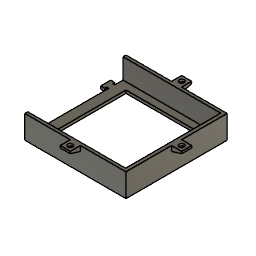
uC podstawa (Autodesk Fusion 360 design; units mm, degrees)
Autodesk Fusion 360 part; units mm, degrees
sketch "Szkic1" plane through (0, 0, 0) normal (0, 0, 1) x (1, 0, 0)
  line L0 (0, 0) -> (100, 0)
  line L1 (100, 0) -> (100, 100)
  line L2 (100, 100) -> (0, 100)
  line L3 (0, 100) -> (0, 0)
  dimension "d1" = 100
  dimension "d2" = 100
  constraint horizontal L0
  constraint vertical L1
  constraint horizontal L2
  constraint vertical L3
  constraint coincident L0.start L3.end
  measures "d1" distance of L0.start L0.end
  measures "d2" distance of L0.start L2.end
extrude "Wyciągnięcie proste1" add sketch "Szkic1" along normal blind 3
sketch "Szkic2" plane through (0, 0, 3) normal (0, 0, 1) x (-1, 0, 0)
  line L0 (0, -100) -> (0, 0)
  line L1 (0, 0) -> (-100, 0)
  line L2 (-100, 0) -> (-100, -100)
  line L3 (-100, -100) -> (0, -100)
  line L4 (-10, -10) -> (-90, -10)
  line L5 (-90, -10) -> (-90, -90)
  line L6 (-90, -90) -> (-10, -90)
  line L7 (-10, -90) -> (-10, -10)
  constraint horizontal L4
  constraint vertical L5
  constraint horizontal L6
  constraint vertical L7
extrude "Wyciągnięcie proste2" cut sketch "Szkic2" against normal blind 3 contours L4 L5 L6 L7
sketch "Szkic3" plane through (0, 0, 3) normal (0, 0, 1) x (-1, 0, 0)
  line L0 (-90, -10) -> (-10, -10)
  line L1 (-10, -10) -> (-10, -90)
  line L2 (-10, -90) -> (-90, -90)
  line L3 (-90, -90) -> (-90, -10)
  line L4 (0, -100) -> (0, 0)
  line L5 (0, 0) -> (-100, 0)
  line L6 (-100, 0) -> (-100, -100)
  line L7 (-100, -100) -> (0, -100)
  line L8 (0, 0) -> (-100, 0)
  line L9 (-100, 0) -> (-100, -3)
  line L10 (-100, -3) -> (0, -3)
  line L11 (0, -3) -> (0, 0)
  line L12 (-100, -3) -> (-96.5907, -3)
  line L13 (-96.5907, -3) -> (-96.5907, -100)
  line L14 (-96.5907, -100) -> (-100, -100)
  line L15 (-100, -100) -> (-100, -3)
  line L16 (-96.5907, -100) -> (0, -100)
  line L17 (0, -100) -> (0, -97)
  line L18 (0, -97) -> (-96.5907, -97)
  line L19 (-96.5907, -97) -> (-96.5907, -100)
  constraint horizontal L8
  constraint vertical L9
  constraint horizontal L10
  constraint vertical L11
  constraint coincident L6 L9.end
  constraint coincident L4.end L5.start
  constraint horizontal L12
  constraint vertical L13
  constraint horizontal L14
  constraint vertical L15
  constraint coincident L7 L13.end
  constraint horizontal L16
  constraint vertical L17
  constraint horizontal L18
  constraint vertical L19
  constraint coincident L4 L17.end
extrude "Wyciągnięcie proste3" add sketch "Szkic3" along normal blind 20 contours L4 L7 L13 L16 L17 L18 L19 | L6 L7 L10 L12 L13 L14 L15 L19 | L4 L5 L6 L8 L9 L10 L11 L12
sketch "Szkic4" plane through (0, 0, 3) normal (0, 0, 1) x (-1, 0, 0)
  line L0 (0, -3) -> (-96.5907, -3)
  line L1 (-96.5907, -3) -> (-96.5907, -97)
  line L2 (-96.5907, -97) -> (0, -97)
  line L3 (0, -97) -> (0, -3)
  line L4 (-90, -10) -> (-10, -10)
  line L5 (-10, -10) -> (-10, -90)
  line L6 (-10, -90) -> (-90, -90)
  line L7 (-90, -90) -> (-90, -10)
  line L8 (0, -97) -> (0, -89)
  line L9 (0, -89) -> (2, -89)
  line L10 (2, -89) -> (2, -91)
  line L11 (2, -91) -> (6, -91)
  line L12 (0, -89) -> (0, -83)
  line L13 (2, -83) -> (2, -81)
  line L14 (2, -81) -> (6, -81)
  line L15 (6, -81) -> (6, -91)
  line L16 (2, -83) -> (0, -83)
  line L17 (0, -83) -> (0, -89.2495)
  constraint coincident L2.end L3.start
  constraint coincident L3 L8.end
  constraint perpendicular L3 L9
  constraint perpendicular L9 L10
  constraint perpendicular L10 L11
  constraint coincident L3 L12.end
  constraint perpendicular L9 L13
  constraint perpendicular L12 L14
  constraint perpendicular L11 L15
  constraint perpendicular L3 L16
  constraint coincident L8 L17.end
extrude "Wyciągnięcie proste4" add sketch "Szkic4" against normal blind 3 contours L3 L9 L10 L11 L12 L13 L14 L15 L16 L17
sketch "Szkic5" plane through (0, 0, 23) normal (0, 0, 1) x (-1, 0, 0)
  line L0 (-100, -100) -> (0, -100)
  line L1 (0, -100) -> (0, -97)
  line L2 (0, -97) -> (-96.5907, -97)
  line L3 (-96.5907, -97) -> (-96.5907, -3)
  line L4 (-96.5907, -3) -> (0, -3)
  line L5 (0, -3) -> (0, 0)
  line L6 (0, 0) -> (-100, 0)
  line L7 (-100, 0) -> (-100, -100)
  line L8 (-45, -100) -> (-55, -100)
  line L9 (-55, -100) -> (-55, -110)
  line L10 (-55, -110) -> (-45, -110)
  line L11 (-45, -110) -> (-45, -100)
  line L12 (-100, -55) -> (-110, -55)
  line L13 (-110, -55) -> (-110, -45)
  line L14 (-110, -45) -> (-100, -45)
  line L15 (-100, -45) -> (-100, -55)
  line L16 (-45, 0) -> (-55, 0)
  line L17 (-55, 0) -> (-55, 10)
  line L18 (-55, 10) -> (-45, 10)
  line L19 (-45, 10) -> (-45, 0)
  constraint horizontal L8
  constraint vertical L9
  constraint horizontal L10
  constraint vertical L11
  constraint coincident L0 L8.start
  constraint horizontal L12
  constraint vertical L13
  constraint horizontal L14
  constraint vertical L15
  constraint coincident L7 L12.start
  constraint horizontal L16
  constraint vertical L17
  constraint horizontal L18
  constraint vertical L19
  constraint coincident L6 L16.start
extrude "Wyciągnięcie proste5" add sketch "Szkic5" against normal blind 2 contours L0 L8 L9 L10 L11 | L7 L12 L13 L14 L15 | L6 L16 L17 L18 L19
sketch "Szkic6" plane through (45, 0, 0) normal (-1, 0, 0) x (0, -1, 0)
  line L0 (10, 23) -> (0, 23)
  line L1 (0, 23) -> (0, 21)
  line L2 (0, 21) -> (10, 21)
  line L3 (10, 21) -> (10, 23)
  line L4 (0, 21) -> (0, 18)
  line L5 (0, 18) -> (10, 21)
  line L6 (0, 21) -> (10, 21)
  constraint coincident L1.end L2.start
  constraint perpendicular L2 L4
  constraint coincident L2.end L3.start
extrude "Wyciągnięcie proste6" add sketch "Szkic6" against normal blind 10 contours L2 L4 L5 L6
sketch "Szkic7" plane through (0, 45, 0) normal (0, -1, 0) x (1, 0, 0)
  line L0 (110, 23) -> (100, 23)
  line L1 (100, 23) -> (100, 21)
  line L2 (100, 21) -> (110, 21)
  line L3 (110, 21) -> (110, 23)
  line L4 (100, 21) -> (100, 18)
  line L5 (100, 18) -> (110, 21)
  line L6 (100, 21) -> (110, 21)
  constraint coincident L1.end L2.start
  constraint perpendicular L2 L4
  constraint coincident L2.end L3.start
extrude "Wyciągnięcie proste7" add sketch "Szkic7" against normal blind 10 contours L2 L4 L5 L6
sketch "Szkic8" plane through (55, 0, 0) normal (1, 0, 0) x (0, 1, 0)
  line L0 (110, 23) -> (100, 23)
  line L1 (100, 23) -> (100, 21)
  line L2 (100, 21) -> (110, 21)
  line L3 (110, 21) -> (110, 23)
  line L4 (100, 21) -> (100, 18)
  line L5 (100, 18) -> (110, 21)
  line L6 (100, 21) -> (110, 21)
  constraint coincident L1.end L2.start
  constraint perpendicular L2 L4
  constraint coincident L2.end L3.start
extrude "Wyciągnięcie proste8" add sketch "Szkic8" against normal blind 10 contours L2 L4 L5 L6
sketch "Szkic9" plane through (0, 0, 23) normal (0, 0, 1) x (-1, 0, 0)
  line L0 (-100, -100) -> (-55, -100)
  line L1 (-55, -100) -> (-55, -110)
  line L2 (-55, -110) -> (-45, -110)
  line L3 (-45, -110) -> (-45, -100)
  line L4 (-45, -100) -> (0, -100)
  line L5 (0, -100) -> (0, -97)
  line L6 (0, -97) -> (-96.5907, -97)
  line L7 (-96.5907, -97) -> (-96.5907, -3)
  line L8 (-96.5907, -3) -> (0, -3)
  line L9 (0, -3) -> (0, 0)
  line L10 (0, 0) -> (-45, 0)
  line L11 (-45, 0) -> (-45, 10)
  line L12 (-45, 10) -> (-55, 10)
  line L13 (-55, 10) -> (-55, 0)
  line L14 (-55, 0) -> (-100, 0)
  line L15 (-100, 0) -> (-100, -45)
  line L16 (-100, -45) -> (-110, -45)
  line L17 (-110, -45) -> (-110, -55)
  line L18 (-110, -55) -> (-100, -55)
  line L19 (-100, -55) -> (-100, -100)
  circle A0 centre (-50, 5) radius 2.5
  circle A1 centre (-105, -50) radius 2.5
  circle A2 centre (-50, -105) radius 2.5
  dimension "d19" = 5
  dimension "d20" = 5
  dimension "d21" = 5
  measures "d19" diameter of A0
  measures "d20" diameter of A1
  measures "d21" diameter of A2
extrude "Wyciągnięcie proste9" cut sketch "Szkic9" against normal blind 2 contours A0 | A1 | A2
